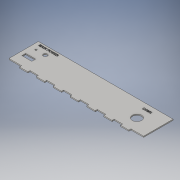
# Autodesk Inventor part: front
Saved by Autodesk Inventor 2016 (Build 200138000, 138)
## iProperties
Created: 2015-08-25
Part Number: front
Material: Generic
Document SubType Name: Modeling
Designer: Chris Gerth
Density: 1 g/cm^3
Appearance: Default
Author: Chris Gerth
Autodesk Inventor part; units mm, degrees
ref_plane "YZ Plane" through (0, 0, 0) normal (1, 0, 0) x (0, 1, 0)
ref_plane "XZ Plane" through (0, 0, 0) normal (0, 1, 0) x (-1, 0, 0)
ref_plane "XY Plane" through (0, 0, 0) normal (0, 0, 1) x (1, 0, 0)
sketch "Sketch1" plane through (0, 0, 0) normal (0, 1, 0) x (-1, 0, 0)
  line L0 (203.2, 31.75) -> (-203.2, 31.75)
  line L1 (-203.2, 31.75) -> (-203.2, -57.15)
  line L2 (-203.2, -57.15) -> (203.2, -57.15)
  line L3 (203.2, -57.15) -> (203.2, 31.75)
  point P0 (0, 0)
  dimension "d0" = 406.4
  dimension "d1" = 88.9
  constraints: 8 end point, 2 parallel, 1 horizontal, 1 perpendicular
  measures "d0" distance of L2.end L1.end
  measures "d1" distance of L1.end L0.end
extrude "Extrusion1" add sketch "Sketch1" along normal blind 3.175
sketch "Sketch2" plane through (0, 3.175, 0) normal (0, 1, 0) x (1, 0, 0)
  line L0 (-203.2, -31.75) -> (203.2, -31.75) projected
  line L1 (-165.1, -31.75) -> (-139.7, -31.75)
  line L2 (-139.7, -31.75) -> (-139.7, -38.1)
  line L3 (-139.7, -38.1) -> (-165.1, -38.1)
  line L4 (-165.1, -38.1) -> (-165.1, -31.75)
  line L5 (-114.3, -31.75) -> (-88.9, -31.75)
  line L6 (-88.9, -31.75) -> (-88.9, -38.1)
  line L7 (-88.9, -38.1) -> (-114.3, -38.1)
  line L8 (-114.3, -38.1) -> (-114.3, -31.75)
  line L9 (-63.5, -31.75) -> (-38.1, -31.75)
  line L10 (-38.1, -31.75) -> (-38.1, -38.1)
  line L11 (-38.1, -38.1) -> (-63.5, -38.1)
  line L12 (-63.5, -38.1) -> (-63.5, -31.75)
  line L13 (-12.7, -31.75) -> (12.7, -31.75)
  line L14 (12.7, -31.75) -> (12.7, -38.1)
  line L15 (12.7, -38.1) -> (-12.7, -38.1)
  line L16 (-12.7, -38.1) -> (-12.7, -31.75)
  line L17 (38.1, -31.75) -> (63.5, -31.75)
  line L18 (63.5, -31.75) -> (63.5, -38.1)
  line L19 (63.5, -38.1) -> (38.1, -38.1)
  line L20 (38.1, -38.1) -> (38.1, -31.75)
  line L21 (88.9, -31.75) -> (114.3, -31.75)
  line L22 (114.3, -31.75) -> (114.3, -38.1)
  line L23 (114.3, -38.1) -> (88.9, -38.1)
  line L24 (88.9, -38.1) -> (88.9, -31.75)
  line L25 (139.7, -31.75) -> (165.1, -31.75)
  line L26 (165.1, -31.75) -> (165.1, -38.1)
  line L27 (165.1, -38.1) -> (139.7, -38.1)
  line L28 (139.7, -38.1) -> (139.7, -31.75)
  point P0 (0, 0)
  dimension "d6" = 50.8
  constraints: 56 end point, 2 horizontal, 2 parallel, 1 collinear, 1 perpendicular, 1 point on line, 47 other
  measures "d6" distance of L1.start L5.start
extrude "Extrusion2" add sketch "Sketch2" against normal blind 3.175
sketch "Sketch3" plane through (-210.3014, 3.175, 39.6064) normal (0, 1, 0) x (1, 0, 0)
  circle A0 centre (355.6026, 45.722) radius 13.97
  point P0 (203.2, 0)
  dimension "d13" = 27.94
  constraints: 1 centre point
  measures "d13" diameter of A0
extrude "Extrusion3" cut sketch "Sketch3" against normal blind 5
sketch "Sketch4" plane through (-216.1175, 3.175, 42.2546) normal (0, 1, 0) x (1, 0, 0)
  line L0 (344.7979, 86.0656) -> (387.5444, 86.0656) construction
  line L1 (387.5444, 86.0656) -> (387.5444, 74.2339) construction
  line L2 (387.5444, 74.2339) -> (344.7979, 74.2339) construction
  line L3 (344.7979, 74.2339) -> (344.7979, 86.0656) construction
  spline S0 degree 2 poles (350.7726, 81.7796) (350.6492, 80.5846) (349.8641, 79.9773) knots 0 0 0 1 1 1
  spline S1 degree 2 poles (349.8641, 79.9773) (349.1431, 79.4193) (347.963, 79.4193) knots 0 0 0 1 1 1
  spline S2 degree 2 poles (347.963, 79.4193) (346.6742, 79.4193) (345.1781, 81.2315) (345.1781, 82.7819) knots 0 0 0 1 2 2 2
  spline S3 degree 2 poles (345.1781, 82.7819) (345.1781, 84.2188) (345.9188, 85.1175) knots 0 0 0 1 1 1
  spline S4 degree 2 poles (345.9188, 85.1175) (346.7039, 86.0656) (348.0865, 86.0656) knots 0 0 0 1 1 1
  spline S5 degree 2 poles (348.0865, 86.0656) (349.2468, 86.0656) (350.743, 84.8212) (350.7726, 83.809) knots 0 0 0 1 2 2 2
  line L4 (350.7726, 83.809) -> (349.5233, 83.809)
  spline S6 degree 2 poles (349.5233, 83.809) (349.474, 84.3126) (348.679, 84.9743) (348.126, 84.9743) knots 0 0 0 1 2 2 2
  spline S7 degree 2 poles (348.126, 84.9743) (347.3507, 84.9743) (346.452, 83.7744) (346.452, 82.7474) knots 0 0 0 1 2 2 2
  spline S8 degree 2 poles (346.452, 82.7474) (346.452, 81.7302) (347.3408, 80.5352) (348.0815, 80.5352) knots 0 0 0 1 2 2 2
  spline S9 degree 2 poles (348.0815, 80.5352) (348.6642, 80.5352) (349.4838, 81.2216) (349.5085, 81.7796) knots 0 0 0 1 2 2 2
  line L5 (349.5085, 81.7796) -> (350.7726, 81.7796)
  spline S10 degree 2 poles (357.5473, 82.7276) (357.5473, 81.2315) (355.8487, 79.4193) (354.4908, 79.4193) knots 0 0 0 1 2 2 2
  spline S11 degree 2 poles (354.4908, 79.4193) (353.0341, 79.4193) (352.2095, 80.4019) knots 0 0 0 1 1 1
  spline S12 degree 2 poles (352.2095, 80.4019) (351.4343, 81.3105) (351.4343, 82.7474) knots 0 0 0 1 1 1
  spline S13 degree 2 poles (351.4343, 82.7474) (351.4343, 84.1299) (352.1651, 85.0385) knots 0 0 0 1 1 1
  spline S14 degree 2 poles (352.1651, 85.0385) (353.0094, 86.0656) (354.5451, 86.0656) knots 0 0 0 1 1 1
  spline S15 degree 2 poles (354.5451, 86.0656) (355.9622, 86.0656) (356.7819, 85.0829) knots 0 0 0 1 1 1
  spline S16 degree 2 poles (356.7819, 85.0829) (357.5473, 84.1596) (357.5473, 82.7276) knots 0 0 0 1 1 1
  spline S17 degree 2 poles (356.2931, 82.7326) (356.2931, 83.7596) (355.3253, 84.9249) (354.471, 84.9249) knots 0 0 0 1 2 2 2
  spline S18 degree 2 poles (354.471, 84.9249) (353.6464, 84.9249) (352.6885, 83.7645) (352.6885, 82.7671) knots 0 0 0 1 2 2 2
  spline S19 degree 2 poles (352.6885, 82.7671) (352.6885, 81.7302) (353.681, 80.5451) (354.5599, 80.5451) knots 0 0 0 1 2 2 2
  spline S20 degree 2 poles (354.5599, 80.5451) (355.3351, 80.5451) (356.2931, 81.7549) (356.2931, 82.7326) knots 0 0 0 1 2 2 2
  line L6 (364.6182, 79.6119) -> (363.3097, 79.6119)
  line L7 (363.3097, 79.6119) -> (363.3097, 84.7669)
  line L8 (363.3097, 84.7669) -> (362.1838, 79.6119)
  line L9 (362.1838, 79.6119) -> (360.8753, 79.6119)
  line L10 (360.8753, 79.6119) -> (359.7446, 84.7422)
  line L11 (359.7446, 84.7422) -> (359.7446, 79.6119)
  line L12 (359.7446, 79.6119) -> (358.4361, 79.6119)
  line L13 (358.4361, 79.6119) -> (358.4361, 85.9619)
  line L14 (358.4361, 85.9619) -> (360.3519, 85.9619)
  line L15 (360.3519, 85.9619) -> (361.5271, 81.1031)
  line L16 (361.5271, 81.1031) -> (362.7171, 85.9619)
  line L17 (362.7171, 85.9619) -> (364.6182, 85.9619)
  line L18 (364.6182, 85.9619) -> (364.6182, 79.6119)
  spline S21 degree 2 poles (370.6324, 81.4833) (370.6324, 80.4908) (369.2301, 79.4094) (367.966, 79.4094) knots 0 0 0 1 2 2 2
  spline S22 degree 2 poles (367.966, 79.4094) (366.8254, 79.4094) (365.502, 80.5056) (365.3983, 81.4932) knots 0 0 0 1 2 2 2
  line L19 (365.3983, 81.4932) -> (366.6624, 81.4932)
  spline S23 degree 2 poles (366.6624, 81.4932) (366.8007, 80.4612) (368.0796, 80.4612) knots 0 0 0 1 1 1
  spline S24 degree 2 poles (368.0796, 80.4612) (368.6721, 80.4612) (369.3782, 80.9056) (369.3782, 81.2907) knots 0 0 0 1 2 2 2
  spline S25 degree 2 poles (369.3782, 81.2907) (369.3782, 81.9968) (368.4993, 82.1647) knots 0 0 0 1 1 1
  line L20 (368.4993, 82.1647) -> (366.9488, 82.461)
  spline S26 degree 2 poles (366.9488, 82.461) (366.3118, 82.5844) (365.5119, 83.4732) (365.5119, 84.0707) knots 0 0 0 1 2 2 2
  spline S27 degree 2 poles (365.5119, 84.0707) (365.5119, 85.0039) (366.7908, 86.0656) (367.9067, 86.0656) knots 0 0 0 1 2 2 2
  spline S28 degree 2 poles (367.9067, 86.0656) (369.1066, 86.0656) (370.4398, 85.0039) (370.4349, 84.0263) knots 0 0 0 1 2 2 2
  line L21 (370.4349, 84.0263) -> (369.2153, 84.0263)
  spline S29 degree 2 poles (369.2153, 84.0263) (369.1856, 84.4904) (368.4499, 85.0286) (367.8574, 85.0286) knots 0 0 0 1 2 2 2
  spline S30 degree 2 poles (367.8574, 85.0286) (366.7414, 85.0286) (366.7414, 84.2089) knots 0 0 0 1 1 1
  spline S31 degree 2 poles (366.7414, 84.2089) (366.7414, 83.6806) (367.4969, 83.5226) knots 0 0 0 1 1 1
  line L22 (367.4969, 83.5226) -> (368.84, 83.2461)
  spline S32 degree 2 poles (368.84, 83.2461) (369.7535, 83.0535) (370.1436, 82.7227) knots 0 0 0 1 1 1
  spline S33 degree 2 poles (370.1436, 82.7227) (370.6324, 82.303) (370.6324, 81.4833) knots 0 0 0 1 1 1
  point P0 (203.2, 0)
  constraints: 2 other
extrude "Extrusion4" cut sketch "Sketch4" against normal blind 1.905
sketch "Sketch5" plane through (-208.4957, 3.175, 40.5353) normal (0, 1, 0) x (1, 0, 0)
  line L0 (17.4181, 47.0558) -> (47.4181, 47.0558)
  line L1 (47.4181, 47.0558) -> (47.4181, 35.5558)
  line L2 (47.4181, 35.5558) -> (17.4181, 35.5558)
  line L3 (17.4181, 35.5558) -> (17.4181, 47.0558)
  point P0 (203.2, 0)
  dimension "d21" = 30
  dimension "d22" = 11.5
  constraints: 8 end point, 2 parallel, 1 horizontal, 1 perpendicular
  measures "d21" distance of L1.end L2.end
  measures "d22" distance of L0.end L1.end
extrude "Extrusion5" cut sketch "Sketch5" against normal blind 5
sketch "Sketch6" plane through (-204.3689, 3.175, 34.8523) normal (0, 1, 0) x (1, 0, 0)
  circle A0 centre (19.1442, 66.6446) radius 2.5
  circle A1 centre (47.3951, 66.6446) radius 6
  point P0 (203.2, 0)
  dimension "d28" = 5
  dimension "d27" = 12
  constraints: 2 centre point
  measures "d28" diameter of A0
  measures "d27" diameter of A1
extrude "Extrusion6" cut sketch "Sketch6" against normal blind 5
sketch "Sketch7" plane through (-201.7656, 3.175, 34.3855) normal (0, 1, 0) x (1, 0, 0)
  line L0 (8.5764, 86.8624) -> (71.354, 86.8624) construction
  line L1 (71.354, 86.8624) -> (71.354, 63.658) construction
  line L2 (71.354, 63.658) -> (8.5764, 63.658) construction
  line L3 (8.5764, 63.658) -> (8.5764, 86.8624) construction
  line L4 (15.3313, 80.4087) -> (14.0227, 80.4087)
  line L5 (14.0227, 80.4087) -> (14.0227, 85.5637)
  line L6 (14.0227, 85.5637) -> (12.8969, 80.4087)
  line L7 (12.8969, 80.4087) -> (11.5884, 80.4087)
  line L8 (11.5884, 80.4087) -> (10.4577, 85.539)
  line L9 (10.4577, 85.539) -> (10.4577, 80.4087)
  line L10 (10.4577, 80.4087) -> (9.1491, 80.4087)
  line L11 (9.1491, 80.4087) -> (9.1491, 86.7587)
  line L12 (9.1491, 86.7587) -> (11.065, 86.7587)
  line L13 (11.065, 86.7587) -> (12.2402, 81.8999)
  line L14 (12.2402, 81.8999) -> (13.4302, 86.7587)
  line L15 (13.4302, 86.7587) -> (15.3313, 86.7587)
  line L16 (15.3313, 86.7587) -> (15.3313, 80.4087)
  line L17 (21.9528, 80.4087) -> (20.6246, 80.4087)
  line L18 (20.6246, 80.4087) -> (20.1752, 81.6826)
  line L19 (20.1752, 81.6826) -> (17.8248, 81.6826)
  line L20 (17.8248, 81.6826) -> (17.3903, 80.4087)
  line L21 (17.3903, 80.4087) -> (16.0571, 80.4087)
  line L22 (16.0571, 80.4087) -> (18.2692, 86.7587)
  line L23 (18.2692, 86.7587) -> (19.7753, 86.7587)
  line L24 (19.7753, 86.7587) -> (21.9528, 80.4087)
  line L25 (19.8642, 82.7739) -> (19.0297, 85.2428)
  line L26 (19.0297, 85.2428) -> (18.2446, 82.7739)
  line L27 (18.2446, 82.7739) -> (19.8642, 82.7739)
  line L28 (23.9823, 80.4087) -> (22.6738, 80.4087)
  line L29 (22.6738, 80.4087) -> (22.6738, 86.7587)
  line L30 (22.6738, 86.7587) -> (23.9823, 86.7587)
  line L31 (23.9823, 86.7587) -> (23.9823, 80.4087)
  line L32 (30.2977, 80.4087) -> (29.0089, 80.4087)
  line L33 (29.0089, 80.4087) -> (26.4413, 84.8477)
  line L34 (26.4413, 84.8477) -> (26.4413, 80.4087)
  line L35 (26.4413, 80.4087) -> (25.1328, 80.4087)
  line L36 (25.1328, 80.4087) -> (25.1328, 86.7587)
  line L37 (25.1328, 86.7587) -> (26.4215, 86.7587)
  line L38 (26.4215, 86.7587) -> (28.9892, 82.4035)
  line L39 (28.9892, 82.4035) -> (28.9892, 86.7587)
  line L40 (28.9892, 86.7587) -> (30.2977, 86.7587)
  line L41 (30.2977, 86.7587) -> (30.2977, 80.4087)
  spline S0 degree 2 poles (38.766, 84.7292) (38.766, 83.8503) (37.7192, 82.6751) (37.0427, 82.6751) knots 0 0 0 1 2 2 2
  line L42 (37.0427, 82.6751) -> (35.2207, 82.6751)
  line L43 (35.2207, 82.6751) -> (35.2207, 80.4087)
  line L44 (35.2207, 80.4087) -> (33.9122, 80.4087)
  line L45 (33.9122, 80.4087) -> (33.9122, 86.7587)
  line L46 (33.9122, 86.7587) -> (36.8995, 86.7587)
  spline S1 degree 2 poles (36.8995, 86.7587) (37.8229, 86.7587) (38.766, 85.6773) (38.766, 84.7292) knots 0 0 0 1 2 2 2
  spline S2 degree 2 poles (37.5019, 84.8082) (37.5019, 85.1983) (37.0822, 85.6674) (36.7119, 85.6674) knots 0 0 0 1 2 2 2
  line L47 (36.7119, 85.6674) -> (35.2207, 85.6674)
  line L48 (35.2207, 85.6674) -> (35.2207, 83.7664)
  line L49 (35.2207, 83.7664) -> (36.7465, 83.7664)
  spline S3 degree 2 poles (36.7465, 83.7664) (37.0575, 83.7664) (37.2847, 84.1071) knots 0 0 0 1 1 1
  spline S4 degree 2 poles (37.2847, 84.1071) (37.5019, 84.4181) (37.5019, 84.8082) knots 0 0 0 1 1 1
  spline S5 degree 2 poles (45.5209, 83.5244) (45.5209, 82.0283) (43.8223, 80.2161) (42.4644, 80.2161) knots 0 0 0 1 2 2 2
  spline S6 degree 2 poles (42.4644, 80.2161) (41.0078, 80.2161) (40.1832, 81.1987) knots 0 0 0 1 1 1
  spline S7 degree 2 poles (40.1832, 81.1987) (39.4079, 82.1073) (39.4079, 83.5442) knots 0 0 0 1 1 1
  spline S8 degree 2 poles (39.4079, 83.5442) (39.4079, 84.9267) (40.1387, 85.8353) knots 0 0 0 1 1 1
  spline S9 degree 2 poles (40.1387, 85.8353) (40.9831, 86.8624) (42.5187, 86.8624) knots 0 0 0 1 1 1
  spline S10 degree 2 poles (42.5187, 86.8624) (43.9359, 86.8624) (44.7556, 85.8797) knots 0 0 0 1 1 1
  spline S11 degree 2 poles (44.7556, 85.8797) (45.5209, 84.9564) (45.5209, 83.5244) knots 0 0 0 1 1 1
  spline S12 degree 2 poles (44.2667, 83.5293) (44.2667, 84.5564) (43.2989, 85.7217) (42.4447, 85.7217) knots 0 0 0 1 2 2 2
  spline S13 degree 2 poles (42.4447, 85.7217) (41.6201, 85.7217) (40.6621, 84.5613) (40.6621, 83.5639) knots 0 0 0 1 2 2 2
  spline S14 degree 2 poles (40.6621, 83.5639) (40.6621, 82.527) (41.6546, 81.3419) (42.5336, 81.3419) knots 0 0 0 1 2 2 2
  spline S15 degree 2 poles (42.5336, 81.3419) (43.3088, 81.3419) (44.2667, 82.5517) (44.2667, 83.5293) knots 0 0 0 1 2 2 2
  line L50 (53.9547, 86.7587) -> (52.1771, 80.4087)
  line L51 (52.1771, 80.4087) -> (51.0019, 80.4087)
  line L52 (51.0019, 80.4087) -> (49.9501, 85.2526)
  line L53 (49.9501, 85.2526) -> (48.9033, 80.4087)
  line L54 (48.9033, 80.4087) -> (47.7281, 80.4087)
  line L55 (47.7281, 80.4087) -> (45.9505, 86.7587)
  line L56 (45.9505, 86.7587) -> (47.3331, 86.7587)
  line L57 (47.3331, 86.7587) -> (48.3108, 82.0036)
  line L58 (48.3108, 82.0036) -> (49.2588, 86.7587)
  line L59 (49.2588, 86.7587) -> (50.6463, 86.7587)
  line L60 (50.6463, 86.7587) -> (51.5944, 81.9493)
  line L61 (51.5944, 81.9493) -> (52.5721, 86.7587)
  line L62 (52.5721, 86.7587) -> (53.9547, 86.7587)
  line L63 (59.4899, 80.4087) -> (54.7447, 80.4087)
  line L64 (54.7447, 80.4087) -> (54.7447, 86.7587)
  line L65 (54.7447, 86.7587) -> (59.3418, 86.7587)
  line L66 (59.3418, 86.7587) -> (59.3418, 85.6674)
  line L67 (59.3418, 85.6674) -> (56.0532, 85.6674)
  line L68 (56.0532, 85.6674) -> (56.0532, 84.2256)
  line L69 (56.0532, 84.2256) -> (59.09, 84.2256)
  line L70 (59.09, 84.2256) -> (59.09, 83.1343)
  line L71 (59.09, 83.1343) -> (56.0532, 83.1343)
  line L72 (56.0532, 83.1343) -> (56.0532, 81.4999)
  line L73 (56.0532, 81.4999) -> (59.4899, 81.4999)
  line L74 (59.4899, 81.4999) -> (59.4899, 80.4087)
  line L75 (65.7659, 80.4087) -> (64.3537, 80.4087)
  spline S16 degree 2 poles (64.3537, 80.4087) (64.1808, 80.8629) (64.1808, 81.1395) knots 0 0 0 1 1 1
  line L76 (64.1808, 81.1395) -> (64.1808, 82.0974)
  spline S17 degree 2 poles (64.1808, 82.0974) (64.1808, 82.4825) (64.0673, 82.6554) knots 0 0 0 1 1 1
  spline S18 degree 2 poles (64.0673, 82.6554) (63.9043, 82.9171) (63.4253, 82.9171) knots 0 0 0 1 1 1
  line L77 (63.4253, 82.9171) -> (61.8749, 82.9171)
  line L78 (61.8749, 82.9171) -> (61.8749, 80.4087)
  line L79 (61.8749, 80.4087) -> (60.5664, 80.4087)
  line L80 (60.5664, 80.4087) -> (60.5664, 86.7587)
  line L81 (60.5664, 86.7587) -> (64.1364, 86.7587)
  spline S19 degree 2 poles (64.1364, 86.7587) (64.7289, 86.7587) (65.1635, 86.3587) knots 0 0 0 1 1 1
  spline S20 degree 2 poles (65.1635, 86.3587) (65.6967, 85.8797) (65.6967, 85.0008) knots 0 0 0 1 1 1
  spline S21 degree 2 poles (65.6967, 85.0008) (65.6967, 83.9787) (64.7635, 83.4652) knots 0 0 0 1 1 1
  spline S22 degree 2 poles (64.7635, 83.4652) (65.44, 83.0998) (65.4597, 82.6455) knots 0 0 0 1 1 1
  line L82 (65.4597, 82.6455) -> (65.5288, 81.095)
  spline S23 degree 2 poles (65.5288, 81.095) (65.5387, 80.8086) (65.7659, 80.6506) knots 0 0 0 1 1 1
  line L83 (65.7659, 80.6506) -> (65.7659, 80.4087)
  spline S24 degree 2 poles (64.4524, 84.9218) (64.4524, 85.6674) (63.7019, 85.6674) knots 0 0 0 1 1 1
  line L84 (63.7019, 85.6674) -> (61.8749, 85.6674)
  line L85 (61.8749, 85.6674) -> (61.8749, 84.0083)
  line L86 (61.8749, 84.0083) -> (63.6772, 84.0083)
  spline S25 degree 2 poles (63.6772, 84.0083) (63.9734, 84.0083) (64.4524, 84.5811) (64.4524, 84.9218) knots 0 0 0 1 2 2 2
  point P0 (203.2, 0)
  constraints: 2 other
extrude "Extrusion7" cut sketch "Sketch7" against normal blind 1.905
equation "\"d16\" = d17"
equation "\"d25\" = d26"
equation "\"d31\" = d28"
equation "\"d17\" = 5"
equation "\"d26\" = 5"
body "Solid1"
